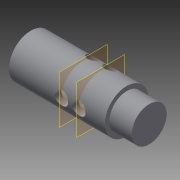
# Autodesk Inventor part: Output SHaft
Saved by Autodesk Inventor 2013 (Build 170138000, 138)
## iProperties
Created: 2013-06-05
Part Number: Output SHaft
Material: Generic
Document SubType Name: Modeling
Designer: mvarma
Density: 1 g/cm^3
Author: mvarma
Autodesk Inventor part; units mm, degrees
ref_plane "YZ Plane" through (0, 0, 0) normal (1, 0, 0) x (0, 1, 0)
ref_plane "XZ Plane" through (0, 0, 0) normal (0, 1, 0) x (-1, 0, 0)
ref_plane "XY Plane" through (0, 0, 0) normal (0, 0, 1) x (1, 0, 0)
sketch "Sketch4" plane through (0, 0, 0) normal (0, 0, 1) x (1, 0, 0)
  line L0 (0, 0) -> (0, 5.5562) construction
  line L1 (0, 5.5562) -> (20.1197, 5.5563)
  line L2 (0, 7.9375) -> (26.1937, 7.9375)
  line L3 (26.1937, 7.9375) -> (26.1937, 6.35)
  line L4 (26.1937, 5.5563) -> (26.1937, 0) construction
  line L5 (26.1937, 0) -> (0, 0) construction
  line L6 (26.1937, 6.35) -> (34.3852, 6.35)
  line L7 (26.1937, 0) -> (31.75, 0) construction
  line L8 (34.3852, 0) -> (34.3852, 6.35)
  line L9 (16.6687, 7.9375) -> (16.6687, 0) construction
  circle A0 centre (16.6687, 7.5565) radius 2.3813 construction
  circle A1 centre (16.6687, 5.4928) radius 2.3813 construction
  circle A2 centre (10.3187, 7.5565) radius 2.3813 construction
  circle A3 centre (10.3187, 5.4928) radius 2.3813 construction
  line L10 (10.3187, 7.9375) -> (10.3187, 0) construction
  line L11 (0, 5.1753) -> (26.1938, 5.1753) construction
  line L12 (8.7312, 5.1753) -> (8.7312, 0) construction
  line L13 (5.5562, 5.1753) -> (5.5562, 0) construction
  line L14 (18.2563, 5.1753) -> (18.2562, 0) construction
  line L15 (21.4313, 5.1753) -> (21.4312, 0) construction
  line L16 (0, 3.1115) -> (26.1937, 3.1115) construction
  line L17 (5.5562, 3.1115) -> (8.7312, 5.1753) construction
  line L18 (18.2563, 5.1753) -> (21.4312, 3.1115) construction
  line L19 (11.9062, 5.1753) -> (11.9062, 0) construction
  line L20 (15.0812, 5.1753) -> (15.0812, 0) construction
  line L21 (11.9062, 5.1753) -> (15.0812, 3.1115) construction
  line L22 (21.4312, 3.3734) -> (29.723, 3.3734)
  line L23 (24.6062, 3.3734) -> (24.6062, 0) construction
  line L24 (21.4312, 3.3734) -> (20.1197, 5.5563)
  line L25 (26.1937, 3.1115) -> (30.9562, 3.1115) construction
  line L26 (30.9562, 3.1115) -> (30.9562, 0) construction
  line L27 (31.75, 3.3734) -> (31.75, 0) construction
  line L28 (31.75, 0) -> (29.723, 3.3734)
  line L29 (0, 7.9375) -> (-1.5875, 7.9375) construction
  line L30 (-1.5875, 7.9375) -> (-1.5875, 3.3734) construction
  line L31 (-1.5875, 3.3734) -> (5.5562, 3.3734) construction
  line L32 (0, 5.5562) -> (0, 7.9375)
  line L33 (0, 7.9375) -> (0, 12.7) construction
  line L34 (20.1197, 5.5563) -> (26.1937, 5.5563) construction
  line L35 (29.723, 3.3734) -> (34.3852, 3.3734) construction
  line L36 (26.1937, 6.35) -> (26.1937, 5.5563) construction
  line L37 (31.75, 0) -> (34.3852, 0)
  line L38 (0, 5.5562) -> (-8.7313, 5.5563)
  line L39 (-8.7313, 5.5563) -> (-8.7313, 7.9375)
  line L40 (-8.7313, 7.9375) -> (0, 7.9375)
  line L41 (-8.7313, 6.35) -> (0, 6.35)
  dimension "d16" = 12.7
  dimension "d17" = 5.5563
  dimension "d18" = 7.9375
  dimension "d19" = 26.1938
  dimension "d20" = 8.1915
  dimension "d21" = 6.35
  dimension "d22" = 9.525
  dimension "d23" = 6.35
  dimension "d24" = 0.381
  dimension "d25" = 0.381
  dimension "d26" = 0.0635
  dimension "d27" = 0.0635
  dimension "d28" = 1.5875
  dimension "d29" = 4.7625
  dimension "d30" = 1.5875
  dimension "d31" = 4.7625
  dimension "d32" = 3.1115
  dimension "d33" = 1.5875
  dimension "d34" = 4.7625
  dimension "d35" = 3.3734
  dimension "d36" = 3.175
  dimension "d37" = 31
  dimension "d38" = 9.525
  dimension "d39" = 9.525
  dimension "d40" = 0.7937
  dimension "d41" = 31
  dimension "d42" = 1.5875
  dimension "d43" = 3.3734
  dimension "d49" = 4.7625
  dimension "d63" = 8.7312
  dimension "d64" = 6.35
  constraints: 82 end point, 33 point on line, 25 perpendicular, 9 vertical, 5 parallel, 4 centre point, 4 coincident, 3 equal radius, 2 collinear, 2 tangent, 1 horizontal, 12 other
  measures "d16" distance of L0.start L33.end
  measures "d17" distance from line of L1 L0.start
  measures "d18" distance from line of L0.start L2
  measures "d19" distance of L2.start L2.end
  measures "d20" distance of L6.start L6.end
  measures "d21" distance of L8.start L6.end
  measures "d22" distance between parallel lines of L3 L9
  measures "d23" distance between parallel lines of L9 L10
  measures "d24" distance from line of L2 A2.centre
  measures "d25" distance from line of L2 A0.centre
  measures "d26" distance from line of L1 A1.centre
  measures "d27" distance from line of L1 A3.centre
  measures "d28" distance between parallel lines of L12 L10
  measures "d29" distance between parallel lines of L13 L10
  measures "d30" distance between parallel lines of L9 L14
  measures "d31" distance between parallel lines of L15 L9
  measures "d32" distance of the line from the sketch origin of L16
  measures "d33" distance between parallel lines of L10 L19
  measures "d34" distance between parallel lines of L10 L20
  measures "d35" distance between parallel lines of L7 L22
  measures "d36" distance between parallel lines of L15 L23
  measures "d37" angle of L15 L24
  measures "d38" distance from line of L23 L21.end
  measures "d39" distance from line of L26 L18.end
  measures "d40" distance between parallel lines of L27 L26
  measures "d41" angle of L27 L28
  measures "d42" distance of L2.start L29.end
  measures "d43" distance of the line from the sketch origin of L31
  measures "d49" diameter of A2
  measures "d63" distance of L39.end L2.start
  measures "d64" distance of the line from the sketch origin of L41
revolve "Revolution1" add sketch "Sketch4" angle 360 about axis through (26.1937, 0, 0) along (-1, 0, 0)
sketch "Sketch5" plane through (0, 0, 0) normal (0, 0, 1) x (1, 0, 0)
  line L0 (26.1937, -7.9375) -> (26.1937, 7.9375) projected
  line L1 (0, 0) -> (26.1937, 0) construction
  circle A0 centre (16.6687, 0) radius 2.4574
  circle A1 centre (10.3187, 0) radius 2.4574
  dimension "d51" = 4.9149
  dimension "d53" = 6.35
  dimension "d54" = 9.525
  dimension "d55" = 4.9149
  constraints: 2 centre point, 2 end point, 2 point on line, 1 midpoint
  measures "d51" diameter of A0
  measures "d53" distance of A1.centre A0.centre
  measures "d54" distance of L1.end A0.centre
  measures "d55" diameter of A1
extrude "Extrusion4" cut sketch "Sketch5" along normal through all
pattern_circular "Circular Pattern2" count 3 over 360 about axis through (-4.3656, 0, 0) along (1, 0, 0) of "Extrusion4"
ref_plane "Work Plane1" through (16.6687, 0, 0) normal (1, 0, 0) x (0, 0, -1)
ref_plane "Work Plane2" through (10.3187, 0, 0) normal (1, 0, 0) x (0, 0, -1)
equation "\"d17\" = d44"
equation "\"d18\" = d45"
equation "\"d24\" = d46"
equation "\"d25\" = d24"
equation "\"d26\" = d47"
equation "\"d27\" = d26"
equation "\"d32\" = d48"
equation "\"d33\" = d28"
equation "\"d34\" = d29"
equation "\"d39\" = d38"
equation "\"d41\" = d37"
equation "\"d43\" = d35"
equation "\"d55\" = d51"
equation "\"d44\" = 5.55625"
equation "\"d45\" = 7.9375"
equation "\"d46\" = 0.381"
equation "\"d47\" = 0.0635"
equation "\"d48\" = 3.1115"
body "Solid2"
